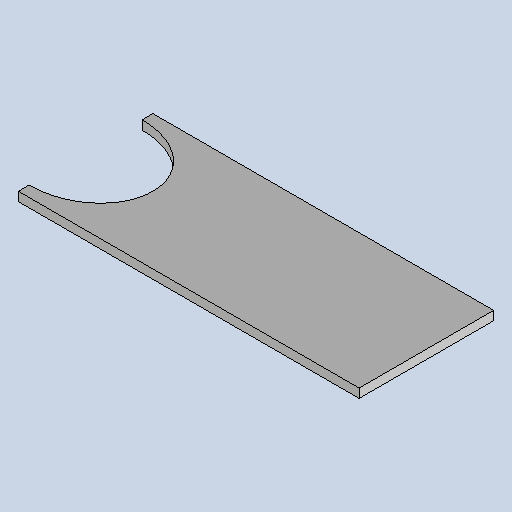
# Autodesk Inventor part: NVPH-344 feeder hose 1
Saved by Autodesk Inventor 2025 (Build 290162010, 162A)
## iProperties
Created: 2024-12-03
Part Number: NVPH-344 feeder hose 1
Material: Generic
Document SubType Name: Sheet Metal
Designer: admin
Density: 1 g/cm^3
Flat Pattern Width: 15 cm
Flat Pattern Length: 38 cm
Flat Pattern Area: 570 cm^2
Sheet Metal Rule: Default_mm
Sheet Metal Width: 150,000 mm
Sheet Metal Length: 380,000 mm
Sheet Metal Area: 57000,000 mm^2
Appearance: Default
Mass: 495.78 g
Surface Area: 1106.68 cm^2
Volume: 495.78 cm^3
Author: user
Autodesk Inventor part; units mm, degrees
ref_plane "YZ Plane" through (0, 0, 0) normal (1, 0, 0) x (0, 1, 0)
ref_plane "XZ Plane" through (0, 0, 0) normal (0, 1, 0) x (-1, 0, 0)
ref_plane "XY Plane" through (0, 0, 0) normal (0, 0, 1) x (1, 0, 0)
sketch "Sketch1" plane through (0, 0, 0) normal (0, 0, 1) x (1, 0, 0)
  ellipse E0 centre (0, 0) end of major axis (75, 0) minor radius 63
  line L0 (0, -63) -> (0, -75)
  line L1 (0, -75) -> (380, -75)
  line L2 (380, -75) -> (380, 75)
  line L3 (380, 75) -> (0, 75)
  line L4 (0, 75) -> (0, 63)
  line L5 (0, 0) -> (380, 0) construction
  point P0 (0, 69)
  dimension "d12" = 75
  dimension "d13" = 63
  dimension "d14" = 150
  dimension "d15" = 380
  measures "d14" distance between parallel lines of L3 L1
  measures "d15" distance of L2.end L3.end
extrude "Plate1" add sketch "Sketch1" along normal blind 10 contours E0 L4 L3 L2 L1 L0
equation "\"d16\" = Thickness"
equation "\"BendReliefDepth\" = 0.5 * Thickness"
equation "\"Thickness\" = 10"
body "Solid2"
